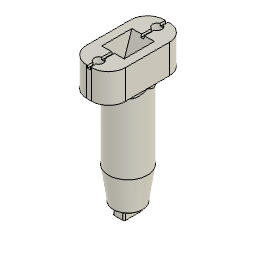
Shroud 0603 straight (Autodesk Fusion 360 design; units mm, degrees)
Autodesk Fusion 360 part; units mm, degrees
sketch "Sketch1" plane through (0, 0, 0) normal (0, 0, 1) x (1, 0, 0)
  circle A0 centre (0, 0) radius 3
  circle A1 centre (0, 0) radius 4
  dimension "d1" = 6
  dimension "d2" = 8
  constraint coincident A0.centre A1.centre
  measures "d1" diameter of A0
  measures "d2" diameter of A1
extrude "Extrude1" add sketch "Sketch1" along normal blind 2
sketch "Sketch2" plane through (0, 0, 2) normal (0, 0, 1) x (-1, 0, 0)
  circle A0 centre (0, 0) radius 3
  circle A1 centre (0, 0) radius 4
  line L0 (-2.3, 1.1) -> (2.3, 1.1)
  line L1 (2.3, 1.1) -> (2.3, -1.1)
  line L2 (2.3, -1.1) -> (-2.3, -1.1)
  line L3 (-2.3, -1.1) -> (-2.3, 1.1)
  line L4 (-2.3, 1.1) -> (2.3, -1.1) construction
  line L5 (2.3, 1.1) -> (-2.3, -1.1) construction
  line L6 (-4, 8) -> (4, 8)
  line L7 (4, 8) -> (4, -8)
  line L8 (4, -8) -> (-4, -8)
  line L9 (-4, -8) -> (-4, 8)
  line L10 (-4, 8) -> (4, -8) construction
  line L11 (4, 8) -> (-4, -8) construction
  dimension "d5" = 4.6
  dimension "d6" = 2.2
  dimension "d7" = 8
  dimension "d8" = 16
  constraint horizontal L0
  constraint perpendicular L0 L1
  constraint parallel L0 L2
  constraint parallel L1 L3
  constraint coincident L4 A0.centre
  constraint coincident L5 A0.centre
  constraint coincident A0.centre A1.centre
  constraint horizontal L6
  constraint perpendicular L6 L7
  constraint parallel L6 L8
  constraint parallel L7 L9
  constraint coincident L10 A0.centre
  constraint coincident L11 A0.centre
  measures "d5" distance of L1.end L2.end
  measures "d6" distance of L0.end L1.end
  measures "d7" distance of L7.end L8.end
  measures "d8" distance of L6.end L7.end
extrude "Extrude2" add sketch "Sketch2" along normal blind 28 contours A0 | A1 | A1 L7 L8 L9 | A1 L6 L7 L9
sketch "Sketch3" plane through (0, 0, 30) normal (0, 0, 1) x (-1, 0, 0)
  line L0 (2.3, -1.1) -> (-2.3, -1.1)
  line L1 (-2.3, -1.1) -> (-2.3, 1.1)
  line L2 (-2.3, 1.1) -> (2.3, 1.1)
  line L3 (2.3, 1.1) -> (2.3, -1.1)
  line L4 (-4, -8) -> (4, -8)
  line L5 (4, -8) -> (4, 8)
  line L6 (4, 8) -> (-4, 8)
  line L7 (-4, 8) -> (-4, -8)
  circle A0 centre (0, -6) radius 0.95
  circle A1 centre (0, 6) radius 0.95
  line L8 (5, 0) -> (-5, 0) construction
  line L9 (0, -10) -> (0, 10) construction
  dimension "d11" = 1.9
  dimension "d12" = 1.9
  dimension "d13" = 6
  dimension "d14" = 6
  constraint perpendicular L3 L8
  constraint perpendicular L6 L9
  measures "d11" diameter of A0
  measures "d12" diameter of A1
  measures "d13" distance of A0.centre L8
  measures "d14" distance of A1.centre L8
fillet "Fillet1" radius 3.5 4 edges at (4, 8, 16) (4, -8, 16) (-4, -8, 16) (-4, 8, 16)
extrude "Extrude3" cut sketch "Sketch3" against normal blind 23 contours A0 | A1
move_face "OffsetFaces1" offset -22 2 faces at (0.0996, -6.6629, 2) (0.0996, 6.6629, 2)
fillet "Fillet2" radius 1 2 edges at (0, 4, 24) (0, -4, 24)
chamfer "Chamfer2" distance 2 distance2 6 2 edges at (0, 1.1, 30) (0, -1.1, 30) measured on face at (0.0237, 2.4176, 30) measured on face at (0.0237, 2.4176, 30)
extrude "Extrude4" cut 1 faces at (3.6518, -0.1987, 0) along direction (0, 0, 1) blind 2
sketch "Sketch4" plane through (0, 0, 2) normal (0, 0, -1) x (1, 0, 0)
  circle A0 centre (0, 0) radius 4
  line L0 (2.3, -1.1) -> (-2.3, -1.1)
  line L1 (-2.3, -1.1) -> (-2.3, 1.1)
  line L2 (-2.3, 1.1) -> (2.3, 1.1)
  line L3 (2.3, 1.1) -> (2.3, -1.1)
  line L4 (-0.7, 1.5) -> (0.7, 1.5)
  line L5 (0.7, 1.5) -> (0.7, -1.5)
  line L6 (0.7, -1.5) -> (-0.7, -1.5)
  line L7 (-0.7, -1.5) -> (-0.7, 1.5)
  line L8 (-0.7, 1.5) -> (0.7, -1.5) construction
  line L9 (0.7, 1.5) -> (-0.7, -1.5) construction
  line L10 (-1.2, 2) -> (1.2, 2)
  line L11 (1.2, 2) -> (1.2, -2)
  line L12 (1.2, -2) -> (-1.2, -2)
  line L13 (-1.2, -2) -> (-1.2, 2)
  line L14 (-1.2, 2) -> (1.2, -2) construction
  line L15 (1.2, 2) -> (-1.2, -2) construction
  dimension "d34" = 1.4
  dimension "d35" = 3
  dimension "d36" = 2.4
  dimension "d37" = 4
  constraint horizontal L4
  constraint perpendicular L4 L5
  constraint parallel L4 L6
  constraint parallel L5 L7
  constraint coincident L8 A0.centre
  constraint coincident L9 A0.centre
  constraint coincident A0.centre origin
  constraint horizontal L10
  constraint perpendicular L10 L11
  constraint parallel L10 L12
  constraint parallel L11 L13
  constraint coincident L14 A0.centre
  constraint coincident L15 A0.centre
  measures "d34" distance of L5.end L6.end
  measures "d35" distance of L4.end L5.end
  measures "d36" distance of L11.end L12.end
  measures "d37" distance of L10.end L11.end
extrude "Extrude5" [suppressed]
extrude "Extrude6" add sketch "Sketch4" along normal blind 0.4 contours A0 | L0 L2 L3 L11 | L0 L1 L2 L13
extrude "Extrude7" add sketch "Sketch4" along normal blind 2 contours L0 L5 L6 L7 L11 L12 L13 | L0 L2 L5 L11 | L2 L4 L5 L7 L10 L11 L13 | L0 L2 L7 L13
fillet "Fillet3" radius 0.3 18 edges at (-0.7, 1.5, 1) (0.7, 1.5, 1) (-1.2, -2, 0.8) (-1.2, 2, 0.8) (-1.2, 0, 1.6) (1.2, -2, 0.8) (0, -2, 1.6) (0, 1.5, 2) (1.2, 0, 1.6) (1.2, 2, 0.8) (0, 2, 1.6) (-0.7, -1.5, 1) (0.7, -1.5, 1) (0, -1.5, 2) (0.7, -1.3, 2) (-0.7, -1.3, 2) (-0.7, 1.3, 2) (0.7, 1.3, 2)
chamfer "Chamfer5" distance 0.2 angle 45 8 edges at (-0.7, 0, 0) (-0.6121, -1.4121, 0) (0, -1.5, 0) (0.6121, -1.4121, 0) (0.7, 0, 0) (0.6121, 1.4121, 0) (0, 1.5, 0) (-0.6121, 1.4121, 0)
sketch "Sketch5" plane through (0, 0, 30) normal (0, 0, 1) x (-1, 0, 0)
  line L0 (2.3, 3.1) -> (2.3, -3.1)
  line L1 (2.3, -3.1) -> (-2.3, -3.1)
  line L2 (-2.3, -3.1) -> (-2.3, 3.1)
  line L3 (-2.3, 3.1) -> (2.3, 3.1)
  circle A0 centre (0, 6) radius 0.95
  circle A1 centre (0, -6) radius 0.95
  arc A2 (0.5, -8) -> (4, -4.5) centre (0.5, -4.5) ccw
  line L4 (4, -4.5) -> (4, 4.5)
  arc A3 (4, 4.5) -> (0.5, 8) centre (0.5, 4.5) ccw
  line L5 (0.5, 8) -> (-0.5, 8)
  arc A4 (-0.5, 8) -> (-4, 4.5) centre (-0.5, 4.5) ccw
  line L6 (-4, 4.5) -> (-4, -4.5)
  arc A5 (-4, -4.5) -> (-0.5, -8) centre (-0.5, -4.5) ccw
  line L7 (-0.5, -8) -> (0.5, -8)
  line L8 (-0.3, 10) -> (0.3, 10)
  line L9 (0.3, 10) -> (0.3, -10)
  line L10 (0.3, -10) -> (-0.3, -10)
  line L11 (-0.3, -10) -> (-0.3, 10)
  line L12 (-0.3, 10) -> (0.3, -10) construction
  line L13 (0.3, 10) -> (-0.3, -10) construction
  dimension "d45" = 0.6
  dimension "d46" = 20
  constraint horizontal L8
  constraint perpendicular L8 L9
  constraint parallel L8 L10
  constraint parallel L9 L11
  constraint coincident L12 origin
  constraint coincident L13 origin
  measures "d45" distance of L9.end L10.end
  measures "d46" distance of L8.end L9.end
extrude "Extrude8" cut sketch "Sketch5" against normal blind 0.5 contours L1 L3 L9 L11 | L3 A0 L9 L11 | L1 A1 L9 L11 | A0 L5 L9 L11 | A1 L7 L9 L11
chamfer "Chamfer6" distance 1 distance2 7 1 edges at (-3.7293, 1.4465, 1.6) measured on face at (-2.3333, 0, 1.6)
fillet "Fillet4" radius 0.5 1 edges at (-2.797, -1.0848, 1.6)
